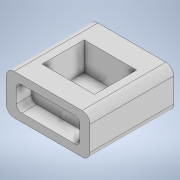
# Autodesk Inventor part: Passenger Section
Saved by Autodesk Inventor 2020 (Build 240168000, 168)
## iProperties
Created: 2020-01-23
Part Number: Passenger Section
Material: Generic
Document SubType Name: Modeling
Designer: cks4a449
Density: 1 g/cm^3
Appearance: Default
Author: cks4a449
Autodesk Inventor part; units mm, degrees
ref_plane "YZ Plane" through (0, 0, 0) normal (1, 0, 0) x (0, 1, 0)
ref_plane "XZ Plane" through (0, 0, 0) normal (0, 1, 0) x (-1, 0, 0)
ref_plane "XY Plane" through (0, 0, 0) normal (0, 0, 1) x (1, 0, 0)
sketch "Sketch1" plane through (0, 0, 0) normal (0, 0, 1) x (1, 0, 0)
  line L0 (7.62, 0) -> (72.644, 0)
  line L1 (80.264, 7.62) -> (80.264, 30.988)
  line L2 (72.644, 38.608) -> (7.62, 38.608)
  line L3 (0, 30.988) -> (0, 7.62)
  arc A0 (7.62, 38.608) -> (0, 30.988) centre (7.62, 30.988) ccw
  arc A1 (0, 7.62) -> (7.62, 0) centre (7.62, 7.62) ccw
  arc A2 (72.644, 0) -> (80.264, 7.62) centre (72.644, 7.62) ccw
  arc A3 (80.264, 30.988) -> (72.644, 38.608) centre (72.644, 30.988) ccw
  point P0 (0, 0)
  point P1 (80.264, 38.608)
  point P2 (80.264, 0)
  point P3 (0, 38.608)
  dimension "d0" = 80.264
  dimension "d1" = 38.608
  dimension "d2" = 7.62
  dimension "d3" = 7.62
  constraints: 8 end point, 8 point on circle, 8 point on line, 8 tangent, 4 centre point, 2 equal radius, 2 parallel, 1 horizontal, 1 perpendicular
  measures "d0" distance of point (0, 38.608) point (80.264, 38.608)
  measures "d1" distance of point (80.264, 38.608) point (80.264, 0)
  measures "d2" radius of A0
  measures "d3" radius of A1
extrude "Extrusion1" add sketch "Sketch1" against normal blind 80.264
sketch "Sketch2" plane through (0, 0, 0) normal (0, 0, 1) x (1, 0, 0)
  line L0 (0, 7.62) -> (0, 30.988) projected
  line L1 (80.264, 30.988) -> (80.264, 7.62) projected
  line L2 (7.62, 38.608) -> (72.644, 38.608) projected
  line L3 (72.644, 0) -> (7.62, 0) projected
  line L4 (14.732, 31.115) -> (65.532, 31.115)
  line L5 (70.612, 26.035) -> (70.612, 12.573)
  line L6 (65.532, 7.493) -> (14.732, 7.493)
  line L7 (9.652, 12.573) -> (9.652, 26.035)
  line L8 (9.652, 31.115) -> (70.612, 7.493) construction
  line L9 (70.612, 31.115) -> (9.652, 7.493) construction
  arc A0 (14.732, 31.115) -> (9.652, 26.035) centre (14.732, 26.035) ccw
  arc A1 (9.652, 12.573) -> (14.732, 7.493) centre (14.732, 12.573) ccw
  arc A2 (65.532, 7.493) -> (70.612, 12.573) centre (65.532, 12.573) ccw
  arc A3 (70.612, 26.035) -> (65.532, 31.115) centre (65.532, 26.035) ccw
  point P0 (0, 0)
  point P1 (40.132, 19.304)
  dimension "d6" = 60.96
  dimension "d7" = 23.622
  dimension "d8" = 5.08
  constraints: 12 end point, 8 point on circle, 8 point on line, 8 tangent, 4 centre point, 3 equal radius, 2 midpoint, 2 parallel, 1 horizontal, 1 perpendicular
  measures "d6" distance of L8.end L9.end
  measures "d7" distance of L9.start L8.end
  measures "d8" radius of A0
extrude "Extrusion2" cut sketch "Sketch2" against normal blind 14.478
sketch "Sketch3" plane through (0, 0, -80.264) normal (0, 0, -1) x (-1, 0, 0)
  line L0 (-72.644, 38.608) -> (-7.62, 38.608) projected
  line L1 (-7.62, 0) -> (-72.644, 0) projected
  line L2 (-80.264, 7.62) -> (-80.264, 30.988) projected
  line L3 (0, 30.988) -> (0, 7.62) projected
  line L4 (-65.532, 7.493) -> (-14.732, 7.493)
  line L5 (-9.652, 12.573) -> (-9.652, 26.035)
  line L6 (-14.732, 31.115) -> (-65.532, 31.115)
  line L7 (-70.612, 26.035) -> (-70.612, 12.573)
  line L8 (-70.612, 7.493) -> (-9.652, 31.115) construction
  line L9 (-9.652, 7.493) -> (-70.612, 31.115) construction
  arc A0 (-65.532, 31.115) -> (-70.612, 26.035) centre (-65.532, 26.035) ccw
  arc A1 (-70.612, 12.573) -> (-65.532, 7.493) centre (-65.532, 12.573) ccw
  arc A2 (-14.732, 7.493) -> (-9.652, 12.573) centre (-14.732, 12.573) ccw
  arc A3 (-9.652, 26.035) -> (-14.732, 31.115) centre (-14.732, 26.035) ccw
  point P0 (0, 0)
  point P1 (-40.132, 19.304)
  dimension "d11" = 60.96
  dimension "d12" = 23.622
  dimension "d13" = 5.08
  constraints: 12 end point, 8 point on circle, 8 point on line, 8 tangent, 4 centre point, 3 equal radius, 2 midpoint, 2 parallel, 1 horizontal, 1 perpendicular
  measures "d11" distance of L9.end L8.end
  measures "d12" distance of L8.end L9.start
  measures "d13" radius of A0
extrude "Extrusion3" cut sketch "Sketch3" against normal blind 14.478
sketch "Sketch4" plane through (7.62, 38.608, 0) normal (0, 1, 0) x (1, 0, 0)
  line L0 (7.366, 59.69) -> (57.658, 59.69)
  line L1 (57.658, 59.69) -> (57.658, 19.304)
  line L2 (57.658, 19.304) -> (7.366, 19.304)
  line L3 (7.366, 19.304) -> (7.366, 59.69)
  line L4 (0, 80.264) -> (65.024, 80.264) projected
  line L5 (-7.62, 0) -> (-7.62, 80.264) projected
  dimension "d16" = 50.292
  dimension "d17" = 40.386
  dimension "d18" = 20.574
  dimension "d19" = 14.986
  constraints: 8 end point, 2 parallel, 1 horizontal, 1 perpendicular
  measures "d16" distance of L1.end L2.end
  measures "d17" distance of L0.end L1.end
  measures "d18" distance between parallel lines of L4 L0
  measures "d19" distance between parallel lines of L5 L3
extrude "Extrusion4" cut sketch "Sketch4" against normal blind 27.178
body "Solid1"
